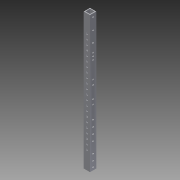
# Autodesk Inventor part: Chassis V1.500 Part4
Saved by Autodesk Inventor 2013 (Build 170138000, 138)
## iProperties
Created: 2013-01-05
Part Number: Chassis V1.500 Part4
Material: Aluminum 6061
Document SubType Name: Modeling
Designer: Moses
Density: 2.71 g/cm^3
Mass: 406.805 g
Surface Area: 997.347 cm^2
Volume: 150.113 cm^3
Author: Moses
Autodesk Inventor part; units mm, degrees
ref_plane "YZ Plane" through (0, 0, 0) normal (1, 0, 0) x (0, 1, 0)
ref_plane "XZ Plane" through (0, 0, 0) normal (0, 1, 0) x (-1, 0, 0)
ref_plane "XY Plane" through (0, 0, 0) normal (0, 0, 1) x (1, 0, 0)
sketch "Sketch1" plane through (0, 0, 0) normal (0, 1, 0) x (-1, 0, 0)
  line L0 (0, 25.4) -> (25.4, 25.4)
  line L1 (25.4, 25.4) -> (25.4, 0)
  line L2 (25.4, 0) -> (0, 0)
  line L3 (0, 0) -> (0, 25.4)
  line L4 (22.225, 22.225) -> (3.175, 22.225)
  line L5 (3.175, 22.225) -> (3.175, 3.175)
  line L6 (3.175, 3.175) -> (22.225, 3.175)
  line L7 (22.225, 3.175) -> (22.225, 22.225)
  dimension "d0" = 25.4
  dimension "d1" = 25.4
  dimension "d2" = 3.175
  constraints: 16 end point, 4 parallel, 2 perpendicular, 1 coincident, 1 horizontal, 3 other
  measures "d0" distance of L1.end L2.end
  measures "d1" distance of L0.end L1.end
  measures "d2" distance between parallel lines of L0 L4
extrude "Extrusion1" add sketch "Sketch1" along normal blind 558.8
sketch "Sketch2" plane through (-25.4, 0, 25.4) normal (0, 0, 1) x (1, 0, 0)
  line L0 (25.4, 0) -> (0, 0) projected
  line L1 (0, 558.8) -> (25.4, 558.8) projected
  line L2 (12.7, 558.8) -> (12.7, 0) construction
  line L3 (12.7, 0) -> (12.7, 13.97) construction
  circle A0 centre (12.7, 13.97) radius 3.302
  circle A1 centre (12.7, 33.6315) radius 3.302
  circle A2 centre (12.7, 53.293) radius 3.302
  circle A3 centre (12.7, 72.9544) radius 3.302
  circle A4 centre (12.7, 92.6159) radius 3.302
  circle A5 centre (12.7, 112.2774) radius 3.302
  circle A6 centre (12.7, 131.9389) radius 3.302
  circle A7 centre (12.7, 151.6004) radius 3.302
  circle A8 centre (12.7, 171.2619) radius 3.302
  circle A9 centre (12.7, 190.9233) radius 3.302
  circle A10 centre (12.7, 210.5848) radius 3.302
  circle A11 centre (12.7, 230.2463) radius 3.302
  circle A12 centre (12.7, 249.9078) radius 3.302
  circle A13 centre (12.7, 269.5693) radius 3.302
  circle A14 centre (12.7, 289.2307) radius 3.302
  circle A15 centre (12.7, 308.8922) radius 3.302
  circle A16 centre (12.7, 328.5537) radius 3.302
  circle A17 centre (12.7, 348.2152) radius 3.302
  circle A18 centre (12.7, 367.8767) radius 3.302
  circle A19 centre (12.7, 387.5381) radius 3.302
  circle A20 centre (12.7, 407.1996) radius 3.302
  circle A21 centre (12.7, 426.8611) radius 3.302
  circle A22 centre (12.7, 446.5226) radius 3.302
  circle A23 centre (12.7, 466.1841) radius 3.302
  circle A24 centre (12.7, 485.8456) radius 3.302
  circle A25 centre (12.7, 505.507) radius 3.302
  circle A26 centre (12.7, 525.1685) radius 3.302
  circle A27 centre (12.7, 544.83) radius 3.302
  dimension "d5" = 13.97
  dimension "d6" = 6.604
  dimension "d7" = 558.8
  dimension "d10" = 19.6615
  constraints: 28 centre point, 4 end point, 2 midpoint, 1 coincident, 1 point on line, 1 vertical, 54 other
  measures "d5" distance of L2.end L3.end
  measures "d6" diameter of A0
  measures "d7" distance of L0.end L1.start
  measures "d10" distance of A0.centre A1.centre
extrude "Extrusion2" cut sketch "Sketch2" against normal through all contours A3 | A4 | A5 | A6 | A7 | A8 | A9 | A10 | A11 | A12 | A13 | A14 | A15 | A16 | A17 | A18 | A19 | A20 | A21 | A22 | A23 | A24
sketch "Sketch3" plane through (-25.4, 0, 0) normal (-1, 0, 0) x (0, 0, 1)
  line L0 (25.4, 0) -> (25.4, 558.8) projected
  line L1 (0, 0) -> (0, 558.8) projected
  line L2 (22.225, 482.5436) -> (22.225, 489.1476) construction
  line L3 (22.225, 344.9132) -> (22.225, 351.5172) construction
  line L4 (22.225, 207.2828) -> (22.225, 213.8868) construction
  line L5 (22.225, 69.6524) -> (22.225, 76.2564) construction
  line L6 (25.4, 485.8456) -> (0, 485.8456) construction
  line L7 (0, 348.2152) -> (25.4, 348.2152) construction
  line L8 (0, 210.5848) -> (25.4, 210.5848) construction
  line L9 (0, 72.9544) -> (25.4, 72.9544) construction
  line L10 (12.7, 498.5456) -> (12.7, 454.0956) construction
  line L11 (12.7, 373.6152) -> (12.7, 322.8152) construction
  line L12 (12.7, 232.8098) -> (12.7, 188.3598) construction
  line L13 (12.7, 104.7044) -> (12.7, 60.2544) construction
  circle A0 centre (12.7, 498.5456) radius 3.302
  circle A1 centre (12.7, 454.0956) radius 3.302
  circle A2 centre (12.7, 373.6152) radius 3.302
  circle A3 centre (12.7, 322.8152) radius 3.302
  circle A4 centre (12.7, 232.8098) radius 3.302
  circle A5 centre (12.7, 188.3598) radius 3.302 construction
  circle A6 centre (12.7, 104.7044) radius 3.302
  circle A7 centre (12.7, 60.2544) radius 3.302
  line L14 (0, 279.4) -> (25.4, 279.4) construction
  line L15 (12.7, 304.8) -> (12.7, 254) construction
  circle A8 centre (12.7, 304.8) radius 3.302
  circle A9 centre (12.7, 254) radius 3.302
  line L16 (25.4, 0) -> (0, 0) projected
  line L17 (0, 558.8) -> (25.4, 558.8) projected
  circle A10 centre (12.7, 546.1) radius 3.302
  line L18 (12.7, 546.1) -> (12.7, 558.8) construction
  line L19 (12.7, 0) -> (12.7, 12.7) construction
  circle A11 centre (12.7, 12.7) radius 3.302
  line L20 (0, 82.4794) -> (25.4, 82.4794) construction
  line L21 (0, 476.3206) -> (25.4, 476.3206) construction
  line L22 (12.7, 12.7) -> (12.7, 34.8544) construction
  circle A12 centre (12.7, 34.8544) radius 3.302
  line L23 (12.7, 104.7044) -> (12.7, 130.1044) construction
  circle A13 centre (12.7, 130.1044) radius 3.302
  line L24 (12.7, 130.1044) -> (12.7, 155.5044) construction
  circle A14 centre (12.7, 155.5044) radius 3.302
  circle A15 centre (12.7, 180.9044) radius 3.302
  line L25 (12.7, 180.9044) -> (12.7, 155.5044) construction
  point P0 (22.225, 485.8456)
  point P1 (22.225, 348.2152)
  point P2 (22.225, 72.9544)
  point P3 (22.225, 210.5848)
  point P4 (12.7, 210.5848)
  point P5 (12.7, 348.2152)
  point P6 (12.7, 279.4)
  point P7 (12.7, 82.4794)
  point P8 (12.7, 476.3206)
  dimension "d17" = 44.45
  dimension "d18" = 50.8
  dimension "d19" = 44.45
  dimension "d20" = 44.45
  dimension "d21" = 6.604
  dimension "d22" = 6.604
  dimension "d23" = 6.604
  dimension "d24" = 6.604
  dimension "d25" = 6.604
  dimension "d26" = 6.604
  dimension "d27" = 6.604
  dimension "d28" = 6.604
  dimension "d31" = 50.8
  dimension "d32" = 6.604
  dimension "d33" = 6.604
  dimension "d40" = 12.7
  dimension "d41" = 6.604
  dimension "d42" = 12.7
  dimension "d43" = 6.604
  dimension "d44" = 9.525
  dimension "d45" = 9.525
  dimension "d60" = 25.4
  dimension "d61" = 6.604
  dimension "d62" = 25.4
  dimension "d63" = 6.604
  dimension "d64" = 25.4
  dimension "d65" = 6.604
  constraints: 36 end point, 16 centre point, 16 midpoint, 14 coincident, 9 collinear, 5 horizontal, 4 point on line, 2 perpendicular, 1 equal radius, 1 parallel, 1 vertical, 16 other
  measures "d17" distance of L10.start L10.end
  measures "d18" distance of L11.start L11.end
  measures "d19" distance of L12.start L12.end
  measures "d20" distance of L13.start L13.end
  measures "d21" diameter of A0
  measures "d22" diameter of A1
  measures "d23" diameter of A2
  measures "d24" diameter of A3
  measures "d25" diameter of A4
  measures "d26" diameter of A5
  measures "d27" diameter of A6
  measures "d28" diameter of A7
  measures "d31" distance of L15.start L15.end
  measures "d32" diameter of A8
  measures "d33" diameter of A9
  measures "d40" distance from line of L17 L18.start
  measures "d41" diameter of A10
  measures "d42" distance of L19.start L19.end
  measures "d43" diameter of A11
  measures "d44" distance between parallel lines of L9 L20
  measures "d45" distance between parallel lines of L6 L21
  measures "d60" distance of L23.start L23.end
  measures "d61" diameter of A13
  measures "d62" distance of L24.start L24.end
  measures "d63" diameter of A14
  measures "d64" distance of L13.end L22.end
  measures "d65" diameter of A12
extrude "Extrusion3" cut sketch "Sketch3" against normal through all contours A0 | A1 | A6 | A7 | A8 | A9 | A10 | A11 | A12 | A13 | A14 | A15
sketch "Sketch4" plane through (0, 0, 25.4) normal (1, 0, 0) x (0, 0, -1)
  circle A0 centre (12.7, 304.8) radius 3.302 projected
  circle A1 centre (12.7, 254) radius 3.302 projected
  line L0 (0, 0) -> (0, 558.8) projected
  line L1 (12.7, 304.8) -> (12.7, 323.85) construction
  line L2 (12.7, 254) -> (12.7, 234.95) construction
  circle A2 centre (12.7, 323.85) radius 3.302
  circle A3 centre (12.7, 234.95) radius 3.302
  line L3 (25.4, 0) -> (0, 0) projected
  line L4 (0, 558.8) -> (25.4, 558.8) projected
  line L5 (12.7, 558.8) -> (12.7, 0) construction
  circle A4 centre (12.7, 431.8) radius 3.302
  circle A5 centre (12.7, 406.4) radius 3.302
  circle A6 centre (12.7, 393.7) radius 3.302
  circle A7 centre (12.7, 419.1) radius 3.302
  circle A8 centre (12.7, 444.5) radius 3.302
  dimension "d46" = 19.05
  dimension "d47" = 19.05
  dimension "d48" = 6.604
  dimension "d49" = 6.604
  dimension "d52" = 6.604
  dimension "d53" = 139.7
  dimension "d54" = 12.7
  dimension "d55" = 12.7
  dimension "d56" = 12.7
  dimension "d57" = 12.7
  constraints: 7 centre point, 6 end point, 5 point on line, 4 equal radius, 2 coincident, 2 midpoint, 1 collinear, 1 parallel
  measures "d46" distance of L1.start L1.end
  measures "d47" distance of L2.start L2.end
  measures "d48" diameter of A2
  measures "d49" diameter of A3
  measures "d52" diameter of A7
  measures "d53" distance from line of L4 A7.centre
  measures "d54" distance of A7.centre A4.centre
  measures "d55" distance of A5.centre A7.centre
  measures "d56" distance of A6.centre A5.centre
  measures "d57" distance of A4.centre A8.centre
extrude "Extrusion4" cut sketch "Sketch4" against normal blind 25.4 contours A2 | A3 | A5 | A6 | A7
equation "\"d19\" = d17"
equation "\"d20\" = d17"
equation "\"d22\" = d21"
equation "\"d23\" = d21"
equation "\"d24\" = d21"
equation "\"d25\" = d21"
equation "\"d26\" = d21"
equation "\"d27\" = d21"
equation "\"d28\" = d21"
equation "\"d31\" = d18"
equation "\"d32\" = d21"
equation "\"d33\" = d21"
equation "\"d41\" = d21"
equation "\"d42\" = d40"
equation "\"d43\" = d21"
equation "\"d45\" = d44"
equation "\"d61\" = d63"
equation "\"d55\" = d54"
equation "\"d56\" = d55"
equation "\"d57\" = d54"
body "Solid1"
